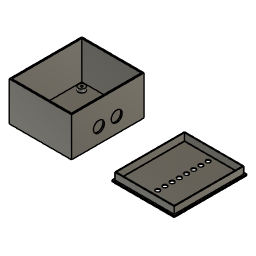
Parking_sensor_enclosure (Autodesk Fusion 360 design; units mm, degrees)
Autodesk Fusion 360 part; units mm, degrees
sketch "Sketch1" plane through (0, 0, 0) normal (0, 0, 1) x (1, 0, 0)
  line L0 (0, 0) -> (91, 0)
  line L1 (91, 0) -> (91, 106)
  line L2 (91, 106) -> (0, 106)
  line L3 (0, 106) -> (0, 0)
  dimension "d1" = 91
  dimension "d2" = 106
  constraint horizontal L0
  constraint vertical L1
  constraint horizontal L2
  constraint vertical L3
  constraint coincident L0.start L3.end
  measures "d1" distance of L0.start L0.end
  measures "d2" distance of L0.start L2.end
extrude "Extrude1" add sketch "Sketch1" along normal blind 55 makes body 1
shell "Shell1" thickness 2 removed faces 1 at (30.3333, 70.6667, 55) on bodies 1
sketch "Sketch2" plane through (0, 0, 2) normal (0, 0, 1) x (-1, 0, 0)
  line L0 (-2, -104) -> (-2, -2)
  line L1 (-2, -2) -> (-89, -2)
  line L2 (-89, -2) -> (-89, -104)
  line L3 (-89, -104) -> (-2, -104)
  circle A0 centre (-78.5, -93.5) radius 5
  circle A1 centre (-78.5, -93.5) radius 1.4
  circle A2 centre (-12.5, -93.5) radius 5
  circle A3 centre (-12.5, -93.5) radius 1.4
  circle A4 centre (-12.5, -12.5) radius 5
  circle A5 centre (-12.5, -12.5) radius 1.4
  circle A6 centre (-78.5, -12.5) radius 5
  circle A7 centre (-78.5, -12.5) radius 1.4
  dimension "d6" = 10
  dimension "d7" = 2.8
  dimension "d8" = 10
  dimension "d9" = 2.8
  dimension "d10" = 10
  dimension "d11" = 2.8
  dimension "d12" = 10
  dimension "d13" = 2.8
  dimension "d100" = 10.5
  dimension "d103" = 10.5
  dimension "d104" = 10.5
  dimension "d105" = 10.5
  dimension "d106" = 10.5
  dimension "d107" = 10.5
  dimension "d108" = 10.5
  dimension "d109" = 10.5
  dimension "d110" = 81
  dimension "d111" = 81
  dimension "d112" = 66
  dimension "d113" = 66
  constraint concentric A0 A1
  constraint concentric A2 A3
  constraint concentric A4 A5
  constraint concentric A6 A7
  measures "d6" diameter of A0
  measures "d7" diameter of A1
  measures "d8" diameter of A2
  measures "d9" diameter of A3
  measures "d10" diameter of A4
  measures "d11" diameter of A5
  measures "d12" diameter of A6
  measures "d13" diameter of A7
  measures "d100" distance of L0 A2.centre
  measures "d103" distance of L3 A2.centre
  measures "d104" distance of L3 A0.centre
  measures "d105" distance of L1 A6.centre
  measures "d106" distance of L2 A6.centre
  measures "d107" distance of L1 A4.centre
  measures "d108" distance of L0 A4.centre
  measures "d109" distance of L2 A0.centre
  measures "d110" distance of A2.centre A4.centre
  measures "d111" distance of A0.centre A6.centre
  measures "d112" distance of A4.centre A6.centre
  measures "d113" distance of A0.centre A2.centre
extrude "Extrude2" add sketch "Sketch2" along normal blind 4 contours A0 | A2 | A4 | A6 bodies 1
extrude "Extrude3" add 4 faces at (8.7238, 93.818, 6) (74.7238, 93.818, 6) (74.7186, 12.7484, 6) (8.7186, 12.7484, 6) along direction (0, 0, 1) blind 1 on bodies 1 bodies 1
sketch "Sketch3" plane through (0, 0, 0) normal (-1, 0, 0) x (0, -1, 0)
  line L0 (-106, 0) -> (0, 0)
  line L1 (0, 0) -> (0, 55)
  line L2 (0, 55) -> (-106, 55)
  line L3 (-106, 55) -> (-106, 0)
  circle A0 centre (-18, 23) radius 8
  line L4 (-2, 2) -> (-2, 55)
  line L5 (-104, 2) -> (-2, 2)
  dimension "d26" = 16
  dimension "d27" = 16
  dimension "d28" = 21
  measures "d26" diameter of A0
  measures "d27" distance of A0.centre L4
  measures "d28" distance of A0.centre L5
extrude "Extrude4" cut sketch "Sketch3" against normal blind 2 contours A0 bodies 1
sketch "Sketch4" plane through (91, 0, 0) normal (1, 0, 0) x (0, 1, 0)
  line L0 (0, 0) -> (106, 0)
  line L1 (106, 0) -> (106, 55)
  line L2 (106, 55) -> (0, 55)
  line L3 (0, 55) -> (0, 0)
  circle A0 centre (40, 22) radius 8
  circle A1 centre (66, 22) radius 8
  line L4 (2, 2) -> (2, 55)
  dimension "d31" = 16
  dimension "d32" = 16
  dimension "d33" = 22
  dimension "d38" = 40
  dimension "d124" = 26
  constraint horizontal A0.centre A1.centre
  measures "d31" diameter of A0
  measures "d32" diameter of A1
  measures "d33" distance of L0 A0.centre
  measures "d38" distance of L3 A0.centre
  measures "d124" distance of A0.centre A1.centre
extrude "Extrude5" cut sketch "Sketch4" against normal blind 2 contours A0 | A1 bodies 1
extrude "Extrude6" add 1 faces at (0.6667, 70, 55) along direction (0, 0, 1) blind 2 on bodies 1 bodies 1
sketch "Sketch5" plane through (0, 0, 2) normal (0, 0, 1) x (-1, 0, 0)
  circle A0 centre (-78.5, -12.5) radius 5
  circle A1 centre (-78.5, -93.5) radius 5
  line L0 (-2, -104) -> (-2, -2)
  line L1 (-2, -2) -> (-89, -2)
  line L2 (-89, -2) -> (-89, -104)
  line L3 (-89, -104) -> (-2, -104)
  circle A2 centre (-12.5, -93.5) radius 5
  circle A3 centre (-12.5, -12.5) radius 5
  line L4 (-150, 0) -> (-241, 0)
  line L5 (-241, 0) -> (-241, -106)
  line L6 (-241, -106) -> (-150, -106)
  line L7 (-150, -106) -> (-150, 0)
  dimension "d44" = 91
  dimension "d45" = 106
  constraint horizontal L4
  constraint vertical L5
  constraint horizontal L6
  constraint vertical L7
  measures "d44" distance of L4.start L4.end
  measures "d45" distance of L4.start L6.end
extrude "Extrude7" add sketch "Sketch5" along normal blind 2 separate body contours L4 L5 L6 L7 makes body 2
sketch "Sketch6" plane through (0, 0, 4) normal (0, 0, 1) x (-1, 0, 0)
  line L0 (-150, -106) -> (-150, 0)
  line L1 (-150, 0) -> (-241, 0)
  line L2 (-241, 0) -> (-241, -106)
  line L3 (-241, -106) -> (-150, -106)
  line L4 (-152.1, -2.1) -> (-238.9, -2.1)
  line L5 (-238.9, -2.1) -> (-238.9, -103.9)
  line L6 (-238.9, -103.9) -> (-152.1, -103.9)
  line L7 (-152.1, -103.9) -> (-152.1, -2.1)
  dimension "d54" = 2.1
  dimension "d55" = 2.1
  dimension "d56" = 2.1
  dimension "d57" = 2.1
  constraint horizontal L4
  constraint vertical L5
  constraint horizontal L6
  constraint vertical L7
  measures "d54" distance of L1 L4
  measures "d55" distance of L2 L5
  measures "d56" distance of L3 L6
  measures "d57" distance of L0 L7
extrude "Extrude8" add sketch "Sketch6" along normal blind 10 contours L4 L5 L6 L7 bodies 2
shell "Shell2" thickness 1 removed faces 1 at (209.9667, 36.0333, 14) on bodies 2
sketch "Sketch7" plane through (0, 0, 3) normal (0, 0, 1) x (-1, 0, 0)
  line L0 (-153.1, -102.9) -> (-153.1, -3.1)
  line L1 (-153.1, -3.1) -> (-237.9, -3.1)
  line L2 (-237.9, -3.1) -> (-237.9, -102.9)
  line L3 (-237.9, -102.9) -> (-153.1, -102.9)
  circle A0 centre (-195.5, -11) radius 3.15
  circle A1 centre (-195.5, -21.5) radius 3.15
  circle A2 centre (-195.5, -32) radius 3.15
  circle A3 centre (-195.5, -42.5) radius 3.15
  circle A4 centre (-195.5, -53) radius 3.15
  circle A5 centre (-195.5, -63.5) radius 3.15
  circle A6 centre (-195.5, -74) radius 3.15
  circle A7 centre (-195.5, -84.5) radius 3.15
  circle A8 centre (-195.5, -95) radius 3.15
  dimension "d61" = 6.3
  dimension "d62" = 6.3
  dimension "d63" = 10.5
  dimension "d68" = 6.3
  dimension "d70" = 6.3
  dimension "d71" = 6.3
  dimension "d72" = 6.3
  dimension "d73" = 6.3
  dimension "d75" = 10.5
  dimension "d76" = 10.5
  dimension "d77" = 10.5
  dimension "d79" = 10.5
  dimension "d80" = 10.5
  dimension "d81" = 7.9
  dimension "d82" = 6.3
  dimension "d83" = 6.3
  dimension "d84" = 10.5
  dimension "d85" = 10.5
  dimension "d87" = 42.4
  dimension "d88" = 42.4
  dimension "d115" = 7.9
  measures "d61" diameter of A0
  measures "d62" diameter of A1
  measures "d63" distance of A0.centre A1.centre
  measures "d68" diameter of A2
  measures "d70" diameter of A3
  measures "d71" diameter of A4
  measures "d72" diameter of A5
  measures "d73" diameter of A6
  measures "d75" distance of A3.centre A4.centre
  measures "d76" distance of A4.centre A5.centre
  measures "d77" distance of A5.centre A6.centre
  measures "d79" distance of A1.centre A2.centre
  measures "d80" distance of A2.centre A3.centre
  measures "d81" distance of L1 A0.centre
  measures "d82" diameter of A7
  measures "d83" diameter of A8
  measures "d84" distance of A6.centre A7.centre
  measures "d85" distance of A7.centre A8.centre
  measures "d87" distance of L0 A0.centre
  measures "d88" distance of L2 A0.centre
  measures "d115" distance of L3 A8.centre
extrude "Extrude11" cut sketch "Sketch7" against normal blind 2 contours A0 | A1 | A2 | A3 | A4 | A5 | A6 | A7 | A8 bodies 2
extrude "Extrude9" [suppressed]
extrude "Extrude10" [suppressed]
